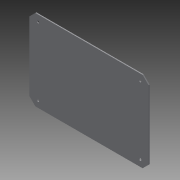
# Autodesk Inventor part: logo na skrzynke z zewnatrz
Saved by Autodesk Inventor 2014 (Build 180170000, 170)
## iProperties
Created: 2018-03-11
Part Number: logo na skrzynke z zewnatrz
Material: Generic
Document SubType Name: Modeling
Designer: HP820
Density: 1 g/cm^3
Appearance: Default
Author: HP820
Autodesk Inventor part; units mm, degrees
ref_plane "YZ Plane" through (0, 0, 0) normal (1, 0, 0) x (0, 1, 0)
ref_plane "XZ Plane" through (0, 0, 0) normal (0, 1, 0) x (-1, 0, 0)
ref_plane "XY Plane" through (0, 0, 0) normal (0, 0, 1) x (1, 0, 0)
sketch "Sketch1" plane through (0, 0, 0) normal (0, 1, 0) x (-1, 0, 0)
  line L0 (-70, 47.5) -> (70, 47.5)
  line L1 (70, 47.5) -> (70, -47.5)
  line L2 (70, -47.5) -> (-70, -47.5)
  line L3 (-70, -47.5) -> (-70, 47.5)
  line L4 (-70, 47.5) -> (70, -47.5) construction
  line L5 (70, 47.5) -> (-70, -47.5) construction
  point P0 (0, 0)
  dimension "d0" = 140
  dimension "d1" = 95
  constraints: 12 end point, 2 midpoint, 2 parallel, 1 horizontal, 1 perpendicular
  measures "d0" distance of L1.end L2.end
  measures "d1" distance of L0.end L1.end
extrude "Extrusion1" add sketch "Sketch1" along normal blind 1.2
sketch "Sketch2" plane through (0, 1.2, 0) normal (0, 1, 0) x (1, 0, 0)
  line L0 (-70, -47.5) -> (70, -47.5) projected
  line L1 (70, -47.5) -> (70, 47.5) projected
  line L2 (-66.1933, 30.2644) -> (66.0954, 30.2644) construction
  line L3 (66.0954, 30.2644) -> (66.0954, -33.1576) construction
  line L4 (66.0954, -33.1576) -> (-66.1933, -33.1576) construction
  line L5 (-66.1933, -33.1576) -> (-66.1933, 30.2644) construction
  line L6 (-63.9633, -15.6357) -> (-63.9633, -32.6621)
  line L7 (-60.6853, -18.1584) -> (-60.6853, -30.1792)
  line L8 (-41.5109, -25.8083) -> (-34.6424, -25.8083)
  line L9 (-19.5119, -23.2049) -> (-19.5119, -21.6888)
  line L10 (-19.5119, -21.6888) -> (-16.6331, -21.6888)
  line L11 (-16.6331, -21.6888) -> (-16.6331, -32.6625)
  line L12 (-16.6331, -32.6625) -> (-19.525, -32.6625)
  line L13 (-19.525, -32.6625) -> (-19.525, -31.473)
  line L14 (-9.1237, -21.6888) -> (-6.2038, -21.6888)
  line L15 (-6.2038, -21.6888) -> (-6.2038, -23.8787)
  line L16 (-6.2038, -23.8787) -> (-9.1237, -23.8787)
  line L17 (-9.1237, -23.8787) -> (-9.1237, -32.6768)
  line L18 (-9.1237, -32.6768) -> (-12.0998, -32.6768)
  line L19 (-12.0998, -32.6768) -> (-12.0998, -23.8787)
  line L20 (-12.0998, -23.8787) -> (-14.2897, -23.8787)
  line L21 (-14.2897, -23.8787) -> (-14.2897, -21.6888)
  line L22 (-14.2897, -21.6888) -> (-12.0998, -21.6888)
  line L23 (-12.0998, -21.6888) -> (-12.0998, -18.3478)
  line L24 (-9.1237, -18.825) -> (-9.1237, -21.6888)
  line L25 (-5.7839, -14.7868) -> (-5.7839, -17.0329)
  line L26 (-6.5688, -32.6768) -> (-3.1435, -32.6768)
  line L27 (-3.1435, -32.6768) -> (-1.0588, -28.2444)
  line L28 (-1.0588, -28.2444) -> (6.8102, -28.2444)
  line L29 (6.8102, -28.2444) -> (9.0695, -32.6768)
  line L30 (9.0695, -32.6768) -> (12.3825, -32.6768)
  line L31 (12.3825, -32.6768) -> (2.9451, -15.0067)
  line L32 (2.9451, -15.0067) -> (-6.5688, -32.6768)
  line L33 (0.366, -25.8083) -> (5.5881, -25.8083)
  line L34 (5.5881, -25.8083) -> (2.977, -20.2569)
  line L35 (2.977, -20.2569) -> (0.366, -25.8083)
  line L36 (14.3742, -15.6525) -> (17.5626, -15.6525)
  line L37 (17.5626, -15.6525) -> (17.5626, -32.6768)
  line L38 (17.5626, -32.6768) -> (14.3742, -32.6768)
  line L39 (14.3742, -32.6768) -> (14.3742, -15.6525)
  line L40 (25.4197, -18.1594) -> (25.4197, -30.1792)
  line L41 (25.4197, -30.1792) -> (29.4051, -30.1792)
  line L42 (25.4197, -18.1594) -> (29.6677, -18.1594)
  line L43 (22.2693, -15.6525) -> (22.2693, -32.6768)
  line L44 (22.2693, -32.6768) -> (29.4051, -32.6768)
  line L45 (22.2693, -15.6525) -> (29.4051, -15.6525)
  line L46 (44.6638, -25.8083) -> (51.534, -25.8083)
  line L47 (51.9647, -28.7122) -> (54.3695, -29.8433)
  line L48 (44.4371, -27.5084) -> (54.6055, -27.5084)
  line L49 (57.6861, -21.6418) -> (57.6861, -32.8183)
  line L50 (57.6861, -32.8183) -> (60.601, -32.8183)
  line L51 (60.601, -32.8183) -> (60.601, -26.8678)
  line L52 (57.6861, -21.6418) -> (60.6064, -21.6418)
  line L53 (60.6064, -21.6418) -> (60.6064, -23.3764)
  line L54 (66.0954, -21.676) -> (65.0828, -23.8289)
  line L55 (-41.7104, -27.5533) -> (-31.5993, -27.5533)
  line L56 (-34.2119, -28.6828) -> (-31.9364, -29.7531)
  line L57 (-15.2472, 28.864) -> (-15.2472, -9.7672)
  line L58 (-15.2472, -9.7672) -> (-1.8118, -9.7672)
  line L59 (-15.2472, 28.864) -> (-1.8118, 28.864)
  line L60 (-12.0859, -0.9518) -> (14.7433, -0.9518)
  line L61 (14.7433, -0.9518) -> (1.3287, 24.165)
  line L62 (1.3287, 24.165) -> (-5.825, 10.8786)
  line L63 (-5.825, 10.8786) -> (0.5297, 10.8786)
  line L64 (0.5297, 10.8786) -> (0.5297, 7.5679)
  line L65 (0.5297, 7.5679) -> (-7.4987, 7.5679)
  line L66 (-7.4987, 7.5679) -> (-12.0859, -0.9518)
  arc A0 (10.0641, 23.831) -> (22.0067, 10.8786) centre (23.783, 24.4984) ccw
  arc A1 (10.0641, 23.831) -> (22.0067, 10.8786) centre (20.8581, 21.8015) ccw
  arc A2 (8.5713, 18.7863) -> (17.5626, 8.9543) centre (19.6677, 19.9066) ccw
  arc A3 (8.5713, 18.7863) -> (17.5626, 8.9543) centre (16.8953, 17.3713) ccw
  arc A4 (12.3478, 26.65) -> (22.3887, 13.7947) centre (29.7614, 29.9022) ccw
  arc A5 (11.939, 26.83) -> (22.4476, 13.3869) centre (24.6266, 25.9191) ccw
  line L67 (-1.8118, 28.864) -> (4.8135, 28.864) construction
  line L68 (4.8135, 28.864) -> (9.6523, 27.8462) construction
  line L69 (9.6523, 27.8462) -> (13.6852, 26.4049) construction
  line L70 (13.6852, 26.4049) -> (17.5626, 23.2133) construction
  line L71 (17.5626, 23.2133) -> (20.8581, 19.0445) construction
  line L72 (20.8581, 19.0445) -> (22.0067, 16.6025) construction
  line L73 (22.0067, 16.6025) -> (22.576, 12.7251) construction
  line L74 (22.576, 12.7251) -> (23.0877, 7.9247) construction
  line L75 (23.0877, 7.9247) -> (21.6611, 2.7429) construction
  line L76 (21.6611, 2.7429) -> (19.6677, -2.7824) construction
  line L77 (19.6677, -2.7824) -> (13.1012, -7.1065) construction
  line L78 (13.1012, -7.1065) -> (9.0695, -9.2598) construction
  line L79 (9.0695, -9.2598) -> (1.6715, -9.7672) construction
  line L80 (1.6715, -9.7672) -> (-1.8118, -9.7672) construction
  spline S0 degree 4 poles (-1.8118, 28.864) (4.8135, 28.864) (9.6523, 27.8462) (13.6852, 26.4049) (17.5626, 23.2133) (20.8581, 19.0445) (22.0067, 16.6025) (22.576, 12.7251) (23.0877, 7.9247) (21.6611, 2.7429) (19.6677, -2.7824) (13.1012, -7.1065) (9.0695, -9.2598) (1.6715, -9.7672) (-1.8118, -9.7672) knots 1 1 1 1 1 2 3 4 5 6 7 8 9 10 11 12 12 12 12 12
  line L81 (-63.9633, -15.6357) -> (-55.565, -15.6357) construction
  line L82 (-55.565, -15.6357) -> (-54.1774, -15.9276) construction
  line L83 (-54.1774, -15.9276) -> (-52.4181, -16.2976) construction
  line L84 (-52.4181, -16.2976) -> (-51.0565, -16.9381) construction
  line L85 (-51.0565, -16.9381) -> (-50.1021, -17.7237) construction
  line L86 (-50.1021, -17.7237) -> (-49.0947, -18.5529) construction
  line L87 (-49.0947, -18.5529) -> (-48.3001, -19.7595) construction
  line L88 (-48.3001, -19.7595) -> (-47.588, -21.2735) construction
  line L89 (-47.588, -21.2735) -> (-47.3662, -22.7838) construction
  line L90 (-47.3662, -22.7838) -> (-47.2397, -24.628) construction
  line L91 (-47.2397, -24.628) -> (-47.5019, -26.5353) construction
  line L92 (-47.5019, -26.5353) -> (-48.1903, -28.4433) construction
  line L93 (-48.1903, -28.4433) -> (-49.35, -30.0676) construction
  line L94 (-49.35, -30.0676) -> (-51.1998, -31.5299) construction
  line L95 (-51.1998, -31.5299) -> (-52.9517, -32.3538) construction
  line L96 (-52.9517, -32.3538) -> (-55.8429, -32.6621) construction
  line L97 (-55.8429, -32.6621) -> (-59.0561, -32.6621) construction
  line L98 (-59.0561, -32.6621) -> (-62.6778, -32.6621) construction
  line L99 (-62.6778, -32.6621) -> (-63.9633, -32.6621) construction
  spline S1 degree 4 poles (-63.9633, -15.6357) (-55.565, -15.6357) (-54.1774, -15.9276) (-52.4181, -16.2976) (-51.0565, -16.9381) (-50.1021, -17.7237) (-49.0947, -18.5529) (-48.3001, -19.7595) (-47.588, -21.2735) (-47.3662, -22.7838) (-47.2397, -24.628) (-47.5019, -26.5353) (-48.1903, -28.4433) (-49.35, -30.0676) (-51.1998, -31.5299) (-52.9517, -32.3538) (-55.8429, -32.6621) (-59.0561, -32.6621) (-62.6778, -32.6621) (-63.9633, -32.6621) knots 1 1 1 1 1 2 3 4 5 6 7 8 9 10 11 12 13 14 15 16 17 17 17 17 17
  line L100 (-60.6853, -18.1584) -> (-58.2186, -18.1584) construction
  line L101 (-58.2186, -18.1584) -> (-55.6727, -18.1584) construction
  line L102 (-55.6727, -18.1584) -> (-53.1129, -18.8632) construction
  line L103 (-53.1129, -18.8632) -> (-51.9914, -20.0564) construction
  line L104 (-51.9914, -20.0564) -> (-51.1648, -21.3116) construction
  line L105 (-51.1648, -21.3116) -> (-50.5799, -22.7186) construction
  line L106 (-50.5799, -22.7186) -> (-50.5799, -24.7797) construction
  line L107 (-50.5799, -24.7797) -> (-51.0357, -26.9464) construction
  line L108 (-51.0357, -26.9464) -> (-51.7576, -28.2872) construction
  line L109 (-51.7576, -28.2872) -> (-53.0834, -29.3352) construction
  line L110 (-53.0834, -29.3352) -> (-54.6403, -30.0676) construction
  line L111 (-54.6403, -30.0676) -> (-56.8465, -30.3027) construction
  line L112 (-56.8465, -30.3027) -> (-60.6853, -30.1792) construction
  spline S2 degree 4 poles (-60.6853, -18.1584) (-58.2186, -18.1584) (-55.6727, -18.1584) (-53.1129, -18.8632) (-51.9914, -20.0564) (-51.1648, -21.3116) (-50.5799, -22.7186) (-50.5799, -24.7797) (-51.0357, -26.9464) (-51.7576, -28.2872) (-53.0834, -29.3352) (-54.6403, -30.0676) (-56.8465, -30.3027) (-60.6853, -30.1792) knots 1 1 1 1 1 2 3 4 5 6 7 8 9 10 11 11 11 11 11
  arc A6 (-34.6424, -25.8083) -> (-41.5109, -25.8083) centre (-38.0766, -26.9577) ccw
  arc A7 (-41.7104, -27.5533) -> (-34.2119, -28.6828) centre (-37.7835, -26.9386) ccw
  line L113 (-31.5993, -27.5533) -> (-31.757, -25.2541) construction
  line L114 (-31.757, -25.2541) -> (-32.2695, -24.1646) construction
  line L115 (-32.2695, -24.1646) -> (-33.865, -22.4669) construction
  line L116 (-33.865, -22.4669) -> (-35.6945, -21.4819) construction
  line L117 (-35.6945, -21.4819) -> (-37.7614, -21.1978) construction
  line L118 (-37.7614, -21.1978) -> (-40.127, -21.4499) construction
  line L119 (-40.127, -21.4499) -> (-42.5978, -22.4469) construction
  line L120 (-42.5978, -22.4469) -> (-44.3932, -24.628) construction
  line L121 (-44.3932, -24.628) -> (-44.9972, -26.822) construction
  line L122 (-44.9972, -26.822) -> (-44.7528, -29.1142) construction
  line L123 (-44.7528, -29.1142) -> (-43.9605, -30.7987) construction
  line L124 (-43.9605, -30.7987) -> (-42.8861, -31.9419) construction
  line L125 (-42.8861, -31.9419) -> (-41.6058, -32.856) construction
  line L126 (-41.6058, -32.856) -> (-39.4115, -33.1576) construction
  line L127 (-39.4115, -33.1576) -> (-36.3229, -33.2571) construction
  line L128 (-36.3229, -33.2571) -> (-34.1341, -32.3471) construction
  line L129 (-34.1341, -32.3471) -> (-32.8931, -31.5299) construction
  line L130 (-32.8931, -31.5299) -> (-32.4154, -30.6427) construction
  line L131 (-32.4154, -30.6427) -> (-31.9364, -29.7531) construction
  spline S3 degree 4 poles (-31.5993, -27.5533) (-31.757, -25.2541) (-32.2695, -24.1646) (-33.865, -22.4669) (-35.6945, -21.4819) (-37.7614, -21.1978) (-40.127, -21.4499) (-42.5978, -22.4469) (-44.3932, -24.628) (-44.9972, -26.822) (-44.7528, -29.1142) (-43.9605, -30.7987) (-42.8861, -31.9419) (-41.6058, -32.856) (-39.4115, -33.1576) (-36.3229, -33.2571) (-34.1341, -32.3471) (-32.8931, -31.5299) (-32.4154, -30.6427) (-31.9364, -29.7531) knots 1 1 1 1 1 2 3 4 5 6 7 8 9 10 11 12 13 14 15 16 17 17 17 17 17
  ellipse E0 centre (-22.889, -27.1842) end of major axis (-22.889, -23.5374) minor radius 3.6468
  line L132 (-19.5119, -23.2049) -> (-20.6683, -21.9744) construction
  line L133 (-20.6683, -21.9744) -> (-22.3863, -21.1978) construction
  line L134 (-22.3863, -21.1978) -> (-24.4254, -21.0684) construction
  line L135 (-24.4254, -21.0684) -> (-26.0717, -21.3116) construction
  line L136 (-26.0717, -21.3116) -> (-27.8804, -22.4056) construction
  line L137 (-27.8804, -22.4056) -> (-29.0058, -24.1646) construction
  line L138 (-29.0058, -24.1646) -> (-29.6136, -26.199) construction
  line L139 (-29.6136, -26.199) -> (-29.5806, -27.6758) construction
  line L140 (-29.5806, -27.6758) -> (-29.2165, -30.3027) construction
  line L141 (-29.2165, -30.3027) -> (-27.3358, -32.117) construction
  line L142 (-27.3358, -32.117) -> (-25.5988, -33.0522) construction
  line L143 (-25.5988, -33.0522) -> (-23.9232, -33.2074) construction
  line L144 (-23.9232, -33.2074) -> (-22.2835, -33.1576) construction
  line L145 (-22.2835, -33.1576) -> (-21.1056, -32.6036) construction
  line L146 (-21.1056, -32.6036) -> (-20.075, -31.9899) construction
  line L147 (-20.075, -31.9899) -> (-19.525, -31.473) construction
  spline S4 degree 4 poles (-19.5119, -23.2049) (-20.6683, -21.9744) (-22.3863, -21.1978) (-24.4254, -21.0684) (-26.0717, -21.3116) (-27.8804, -22.4056) (-29.0058, -24.1646) (-29.6136, -26.199) (-29.5806, -27.6758) (-29.2165, -30.3027) (-27.3358, -32.117) (-25.5988, -33.0522) (-23.9232, -33.2074) (-22.2835, -33.1576) (-21.1056, -32.6036) (-20.075, -31.9899) (-19.525, -31.473) knots 1 1 1 1 1 2 3 4 5 6 7 8 9 10 11 12 13 14 14 14 14 14
  line L148 (-12.0998, -18.3478) -> (-11.9624, -16.8638) construction
  line L149 (-11.9624, -16.8638) -> (-11.7148, -16.0348) construction
  line L150 (-11.7148, -16.0348) -> (-11.0998, -15.0736) construction
  line L151 (-11.0998, -15.0736) -> (-10.6181, -14.7868) construction
  line L152 (-10.6181, -14.7868) -> (-10.2466, -14.5168) construction
  line L153 (-10.2466, -14.5168) -> (-8.7471, -14.309) construction
  line L154 (-8.7471, -14.309) -> (-7.3831, -14.309) construction
  line L155 (-7.3831, -14.309) -> (-5.7839, -14.7868) construction
  spline S5 degree 4 poles (-12.0998, -18.3478) (-11.9624, -16.8638) (-11.7148, -16.0348) (-11.0998, -15.0736) (-10.6181, -14.7868) (-10.2466, -14.5168) (-8.7471, -14.309) (-7.3831, -14.309) (-5.7839, -14.7868) knots 1 1 1 1 1 2 3 4 5 6 6 6 6 6
  line L156 (-9.1237, -18.825) -> (-9.0218, -17.7237) construction
  line L157 (-9.0218, -17.7237) -> (-8.633, -16.8638) construction
  line L158 (-8.633, -16.8638) -> (-7.6638, -16.4079) construction
  line L159 (-7.6638, -16.4079) -> (-6.4782, -16.4079) construction
  line L160 (-6.4782, -16.4079) -> (-5.7839, -17.0329) construction
  spline S6 degree 4 poles (-9.1237, -18.825) (-9.0218, -17.7237) (-8.633, -16.8638) (-7.6638, -16.4079) (-6.4782, -16.4079) (-5.7839, -17.0329) knots 1 1 1 1 1 2 3 3 3 3 3
  arc A8 (29.4051, -30.1792) -> (29.6677, -18.1594) centre (29.6677, -24.1721) ccw
  arc A9 (29.4051, -32.6768) -> (29.4051, -15.6525) centre (30.3874, -24.1646) ccw
  arc A10 (51.534, -25.8083) -> (44.6638, -25.8083) centre (48.0989, -26.8811) ccw
  line L161 (54.6055, -27.5084) -> (54.6055, -25.1818) construction
  line L162 (54.6055, -25.1818) -> (53.062, -22.5897) construction
  line L163 (53.062, -22.5897) -> (51.1801, -21.3856) construction
  line L164 (51.1801, -21.3856) -> (47.725, -20.9107) construction
  line L165 (47.725, -20.9107) -> (44.4725, -21.676) construction
  line L166 (44.4725, -21.676) -> (41.7485, -23.8787) construction
  line L167 (41.7485, -23.8787) -> (41.4589, -25.9852) construction
  line L168 (41.4589, -25.9852) -> (41.1562, -29.2554) construction
  line L169 (41.1562, -29.2554) -> (42.7949, -31.2099) construction
  line L170 (42.7949, -31.2099) -> (44.6254, -33.1576) construction
  line L171 (44.6254, -33.1576) -> (48.6216, -33.1576) construction
  line L172 (48.6216, -33.1576) -> (52.7563, -32.5846) construction
  line L173 (52.7563, -32.5846) -> (54.3695, -29.8433) construction
  spline S7 degree 4 poles (54.6055, -27.5084) (54.6055, -25.1818) (53.062, -22.5897) (51.1801, -21.3856) (47.725, -20.9107) (44.4725, -21.676) (41.7485, -23.8787) (41.4589, -25.9852) (41.1562, -29.2554) (42.7949, -31.2099) (44.6254, -33.1576) (48.6216, -33.1576) (52.7563, -32.5846) (54.3695, -29.8433) knots 1 1 1 1 1 2 3 4 5 6 7 8 9 10 11 11 11 11 11
  line L174 (60.601, -26.8678) -> (60.7369, -25.3997) construction
  line L175 (60.7369, -25.3997) -> (61.4406, -24.2041) construction
  line L176 (61.4406, -24.2041) -> (62.1499, -23.5374) construction
  line L177 (62.1499, -23.5374) -> (63.092, -23.3158) construction
  line L178 (63.092, -23.3158) -> (64.044, -23.3158) construction
  line L179 (64.044, -23.3158) -> (64.7634, -23.641) construction
  line L180 (64.7634, -23.641) -> (65.0828, -23.8289) construction
  spline S8 degree 4 poles (60.601, -26.8678) (60.7369, -25.3997) (61.4406, -24.2041) (62.1499, -23.5374) (63.092, -23.3158) (64.044, -23.3158) (64.7634, -23.641) (65.0828, -23.8289) knots 1 1 1 1 1 2 3 4 5 5 5 5 5
  line L181 (44.4371, -27.5084) -> (44.4887, -29.2105) construction
  line L182 (44.4887, -29.2105) -> (45.5743, -30.1877) construction
  line L183 (45.5743, -30.1877) -> (46.9904, -31.2382) construction
  line L184 (46.9904, -31.2382) -> (48.3266, -30.7823) construction
  line L185 (48.3266, -30.7823) -> (50.3157, -30.722) construction
  line L186 (50.3157, -30.722) -> (51.0655, -29.7111) construction
  line L187 (51.0655, -29.7111) -> (51.9647, -28.7122) construction
  spline S9 degree 4 poles (44.4371, -27.5084) (44.4887, -29.2105) (45.5743, -30.1877) (46.9904, -31.2382) (48.3266, -30.7823) (50.3157, -30.722) (51.0655, -29.7111) (51.9647, -28.7122) knots 1 1 1 1 1 2 3 4 5 5 5 5 5
  line L188 (60.6064, -23.3764) -> (61.1407, -22.2406) construction
  line L189 (61.1407, -22.2406) -> (62.0413, -21.3941) construction
  line L190 (62.0413, -21.3941) -> (63.6358, -21.1731) construction
  line L191 (63.6358, -21.1731) -> (65.2728, -21.1235) construction
  line L192 (65.2728, -21.1235) -> (66.0908, -21.6429) construction
  spline S10 degree 4 poles (60.6064, -23.3764) (61.1407, -22.2406) (62.0413, -21.3941) (63.6358, -21.1731) (65.2728, -21.1235) (66.0908, -21.6429) knots 1 1 1 1 1 2 3 3 3 3 3
  line L193 (66.0908, -21.6429) -> (66.0954, -21.676)
  point P0 (0, 0)
  constraints: 124 end point, 79 parallel, 61 perpendicular, 22 point on circle, 11 centre point, 5 point on line, 2 collinear, 1 tangent, 1 vertical, 41 other
extrude "Extrusion2" add sketch "Sketch2" along normal blind 1.2 contours S1 L6 | L9 L10 L11 L12 L13 S4 | L14 L15 L16 L17 L18 L19 L20 L21 L22 L23 S5 L25 S6 L24 | L32 L31 L30 L29 L28 L27 L26 | L36 L37 L38 L39 | L45 A9 L44 L43 | L47 S7 L48 S9 | L52 L53 S10 L193 L54 S8 L51 L50 L49 | A7 L56 S3 L55 | L59 S0 A5 L58 L57 | S0 A4
sketch "Sketch3" plane through (0, 1.2, 0) normal (0, 1, 0) x (1, 0, 0)
  line L0 (-60, -40) -> (60, -40)
  line L1 (60, -40) -> (60, 40)
  line L2 (60, 40) -> (-60, 40)
  line L3 (-60, 40) -> (-60, -40)
  line L4 (-60, -40) -> (60, 40) construction
  line L5 (60, -40) -> (-60, 40) construction
  circle A0 centre (-60, 40) radius 1.5
  circle A1 centre (60, 40) radius 1.5
  circle A2 centre (60, -40) radius 1.5
  circle A3 centre (-60, -40) radius 1.5
  point P0 (0, 0)
  dimension "d40" = 120
  dimension "d41" = 80
  dimension "d42" = 3
  dimension "d43" = 3
  dimension "d44" = 3
  constraints: 12 end point, 4 centre point, 4 coincident, 2 midpoint, 2 parallel, 1 horizontal, 1 perpendicular
  measures "d40" distance of L2.end L1.end
  measures "d41" distance of L1.end L0.end
  measures "d42" diameter of A0
  measures "d43" diameter of A1
  measures "d44" diameter of A3
extrude "Extrusion3" cut sketch "Sketch3" against normal blind 17.05 contours L3 A3 L0 | L0 A3 L3 | A2 L1 L0 | L0 L1 A2 | A0 L2 L3 | L3 L2 A0 | A1 L2 L1 | L1 L2 A1
chamfer "Chamfer1" distance 7 angle 45 4 edges at (70, 0.6, -47.5) (-70, 0.6, -47.5) (-70, 0.6, 47.5) (70, 0.6, 47.5)
body "Solid1"
